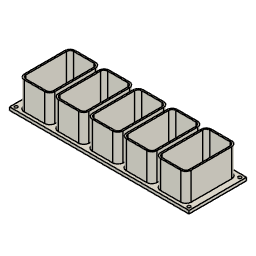
Skittle boxes (Autodesk Fusion 360 design; units mm, degrees)
Autodesk Fusion 360 part; units mm, degrees
sketch "Sketch1" plane through (0, 0, 0) normal (0, 1, 0) x (1, 0, 0) in component "Box"
  line L0 (-15, 25) -> (15, 25)
  line L1 (15, 25) -> (15, -25)
  line L2 (15, -25) -> (-15, -25)
  line L3 (-15, -25) -> (-15, 25)
  line L4 (-15, -25) -> (15, 25) construction
  dimension "d1" = 30
  dimension "d2" = 50
  constraint horizontal L0
  constraint vertical L1
  constraint horizontal L2
  constraint vertical L3
  constraint midpoint origin L4
  measures "d1" distance of L1.end L2.end
  measures "d2" distance of L0.start L2.end
extrude "Extrude1" add sketch "Sketch1" along normal blind 30 makes body 1 in component "Box"
fillet "Fillet1" radius 5 4 edges at (15, 15, 25) (-15, 15, 25) (15, 15, -25) (-15, 15, -25) on bodies 1 in component "Box"
fillet "Fillet2" radius 0.5 8 edges at (13.5355, 0, -23.5355) (0, 0, -25) (-13.5355, 0, -23.5355) (-15, 0, 0) (-13.5355, 0, 23.5355) (0, 0, 25) (13.5355, 0, 23.5355) (15, 0, 0) on bodies 1 in component "Box"
shell "Shell1" thickness 1.5 removed faces 1 at (-5, 30, 6.6667) on bodies 1 in component "Box"
sketch "Sketch1 (2)" plane through (0, 0, 0) normal (0, 1, 0) x (1, 0, 0) in component "Frame"
  line L0 (-88.25, 28.25) -> (88.25, 28.25)
  line L1 (88.25, 28.25) -> (88.25, -28.25)
  line L2 (88.25, -28.25) -> (-88.25, -28.25)
  line L3 (-88.25, -28.25) -> (-88.25, 28.25)
  line L4 (-82.25, 25.25) -> (-51.75, 25.25)
  line L5 (-51.75, 25.25) -> (-51.75, -25.25)
  line L6 (-51.75, -25.25) -> (-82.25, -25.25)
  line L7 (-82.25, -25.25) -> (-82.25, 25.25)
  line L8 (-82.25, -25.25) -> (-51.75, 25.25) construction
  line L9 (-18.25, 25.25) -> (-18.25, -25.25)
  line L10 (-18.25, -25.25) -> (-48.75, -25.25)
  line L11 (-48.75, -25.25) -> (-48.75, 25.25)
  line L12 (-48.75, 25.25) -> (-18.25, 25.25)
  line L13 (15.25, 25.25) -> (15.25, -25.25)
  line L14 (15.25, -25.25) -> (-15.25, -25.25)
  line L15 (-15.25, -25.25) -> (-15.25, 25.25)
  line L16 (-15.25, 25.25) -> (15.25, 25.25)
  line L17 (48.75, 25.25) -> (48.75, -25.25)
  line L18 (48.75, -25.25) -> (18.25, -25.25)
  line L19 (18.25, -25.25) -> (18.25, 25.25)
  line L20 (18.25, 25.25) -> (48.75, 25.25)
  line L21 (82.25, 25.25) -> (82.25, -25.25)
  line L22 (82.25, -25.25) -> (51.75, -25.25)
  line L23 (51.75, -25.25) -> (51.75, 25.25)
  line L24 (51.75, 25.25) -> (82.25, 25.25)
  line L25 (-82.25, -25.25) -> (82.25, 25.25) construction
  line L26 (88.25, -28.25) -> (-88.25, 28.25) construction
  line L27 (85, -25) -> (-85, -25) construction
  line L28 (-85, -25) -> (-85, 25) construction
  line L29 (-85, 25) -> (85, 25) construction
  line L30 (85, 25) -> (85, -25) construction
  line L31 (85, 0) -> (-85, 0) construction
  circle A0 centre (85, -25) radius 1.5
  circle A1 centre (85, 25) radius 1.5
  circle A2 centre (-85, 25) radius 1.5
  circle A3 centre (-85, -25) radius 1.5
  dimension "d10" = 30.5
  dimension "d11" = 50.5
  dimension "d14" = 33.5
  dimension "d15" = 0
  dimension "d16" = 3
  dimension "d19" = 6
  dimension "d24" = 170
  dimension "d25" = 50
  dimension "d26" = 3
  dimension "d27" = 3
  dimension "d28" = 3
  dimension "d29" = 3
  constraint horizontal L0
  constraint vertical L1
  constraint horizontal L2
  constraint vertical L3
  constraint horizontal L4
  constraint vertical L5
  constraint horizontal L6
  constraint vertical L7
  constraint midpoint origin L26
  constraint midpoint origin L25
  constraint horizontal L27
  constraint vertical L28
  constraint horizontal L29
  constraint vertical L30
  constraint midpoint L30 L31.start
  constraint midpoint L28 L31.end
  constraint midpoint origin L31
  constraint coincident L27.start L30.end
  constraint coincident L29.end L30.start
  constraint coincident L28.end L29.start
  constraint coincident L27.end L28.start
  measures "d10" distance of L4.start L4.end
  measures "d11" distance of L4.start L6.end
  measures "d16" distance of L0 L24
  measures "d19" distance of L1 L21
  measures "d24" distance of L27.start L27.end
  measures "d25" distance of L27.start L29.end
  measures "d26" diameter of A0
  measures "d27" diameter of A1
  measures "d28" diameter of A2
  measures "d29" diameter of A3
extrude "Extrude1'" add sketch "Sketch1 (2)" along normal blind 3 separate body makes body 2 in component "Frame"
fillet "Fillet1'" radius 5.25 20 edges at (18.25, 1.5, -25.25) (51.75, 1.5, -25.25) (-15.25, 1.5, -25.25) (-48.75, 1.5, -25.25) (-82.25, 1.5, -25.25) (-51.75, 1.5, -25.25) (-18.25, 1.5, -25.25) (15.25, 1.5, -25.25) (48.75, 1.5, -25.25) (82.25, 1.5, -25.25) (82.25, 1.5, 25.25) (51.75, 1.5, 25.25) (18.25, 1.5, 25.25) (48.75, 1.5, 25.25) (15.25, 1.5, 25.25) (-51.75, 1.5, 25.25) (-18.25, 1.5, 25.25) (-15.25, 1.5, 25.25) (-48.75, 1.5, 25.25) (-82.25, 1.5, 25.25) on bodies 2 in component "Frame"
pattern_linear "00000000-0000-0000-0000-000000000000" [suppressed]
component "Frame" placed x (1, 0, 0) y (0, 1, 0) z (0, 0, 1) at (0, 0, 0)
component "Box" placed x (1, 0, 0) y (0, 1, 0) z (0, 0, 1) at (-67, 0, 0)
component "Box" placed x (1, 0, 0) y (0, 1, 0) z (0, 0, 1) at (-33.5, 0, 0)
component "Box" placed x (1, 0, 0) y (0, 1, 0) z (0, 0, 1) at (0, 0, 0)
component "Box" placed x (1, 0, 0) y (0, 1, 0) z (0, 0, 1) at (33.5, 0, 0)
component "Box" placed x (1, 0, 0) y (0, 1, 0) z (0, 0, 1) at (67, 0, 0)
equation "d1 = BoxWidth"
equation "d10 = BoxWidth + 0.5 mm"
equation "d14 = d10 + 3 mm"
equation "d27 = d26"
equation "d28 = d26"
equation "d29 = d26"
equation "BoxWidth = 30 mm"
